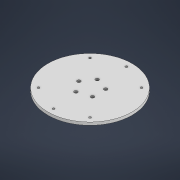
# Autodesk Inventor part: Bottom
Saved by Autodesk Inventor 2021 (Build 250183000, 183)
## iProperties
Created: 2022-09-26
Part Number: Bottom
Material: Ogólny
Document SubType Name: Modeling
Designer: MicnedSQ
Density: 1 g/cm^3
Appearance: Domyślna
Author: MicnedSQ
## iProperties of the stored document _Drukowanie 3D.ipt
Created: 2022-10-01
Part Number: _Drukowanie 3D
Material: Ogólny
Document SubType Name: Modeling
Designer: MicnedSQ
Density: 1 g/cm^3
Appearance: Domyślna
Author: MicnedSQ
Autodesk Inventor part; units mm, degrees
ref_plane "YZ Plane" through (0, 0, 0) normal (1, 0, 0) x (0, 1, 0)
ref_plane "XZ Plane" through (0, 0, 0) normal (0, 1, 0) x (-1, 0, 0)
ref_plane "XY Plane" through (0, 0, 0) normal (0, 0, 1) x (1, 0, 0)
sketch "Szkic1" plane through (0, 0, 0) normal (0, 1, 0) x (-1, 0, 0)
  circle A0 centre (0, 0) radius 25
  dimension "d0" = 50
  constraints: 1 centre point, 1 coincident
  measures "d0" diameter of A0
extrude "Wyciągnięcie proste1" add sketch "Szkic1" along normal blind 2
sketch "Szkic2" plane through (0, 2, 0) normal (0, 1, 0) x (1, 0, 0)
  circle A0 centre (0, 0) radius 75
  dimension "d3" = 150
  constraints: 1 centre point, 1 coincident
  measures "d3" diameter of A0
extrude "Wyciągnięcie proste2" add sketch "Szkic2" along normal blind 5
sketch "Szkic3" plane through (0, 7, 0) normal (0, 1, 0) x (1, 0, 0)
  circle A0 centre (-20, 0) radius 3
  point P0 (0, 0)
  dimension "d6" = 6
  dimension "d7" = 20
  constraints: 1 centre point
  measures "d6" diameter of A0
  measures "d7" distance of point (0, 0) A0.centre
extrude "Wyciągnięcie proste3" cut sketch "Szkic3" against normal blind 4
sketch "Szkic4" plane through (-20, 3, 0) normal (0, 1, 0) x (1, 0, 0)
  circle A0 centre (0, 0) radius 3 projected
  circle A1 centre (0, 0) radius 1.75
  point P0 (20, 0)
  dimension "d10" = 3.5
  constraints: 1 centre point, 1 coincident
  measures "d10" diameter of A1
extrude "Wyciągnięcie proste4" cut sketch "Szkic4" against normal through all contours A1
pattern_circular "Szyk kołowy1" count 5 over 360 about axis through (0, 0, 0) along (0, 1, 0) of "Wyciągnięcie proste3", "Wyciągnięcie proste4"
sketch "Szkic5" plane through (0, 7, 0) normal (0, 1, 0) x (1, 0, 0)
  circle A0 centre (0, 65) radius 1.95
  point P0 (0, 0)
  dimension "d16" = 3.9
  dimension "d17" = 65
  constraints: 1 centre point
  measures "d16" diameter of A0
  measures "d17" distance of point (0, 0) A0.centre
extrude "Wyciągnięcie proste5" cut sketch "Szkic5" against normal blind 4
pattern_circular "Szyk kołowy2" count 8 over 360 about axis through (0, 2, 0) along (0, 1, 0) of "Wyciągnięcie proste5" skipped copies 3 7
